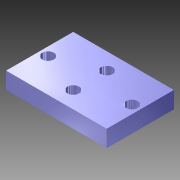
# Autodesk Inventor part: tapa polea x
Saved by Autodesk Inventor 2012 SP2 (Build 160219200, 219)
## iProperties
Created: 2014-07-05
Part Number: tapa polea x
Material: Default
Document SubType Name: Modeling
Designer: Principal
Density: 1 g/cm^3
Author: Principal
Autodesk Inventor part; units mm, degrees
ref_plane "YZ Plane" through (0, 0, 0) normal (1, 0, 0) x (0, 1, 0)
ref_plane "XZ Plane" through (0, 0, 0) normal (0, 1, 0) x (-1, 0, 0)
ref_plane "XY Plane" through (0, 0, 0) normal (0, 0, 1) x (1, 0, 0)
sketch "Boceto1" plane through (0, 0, 0) normal (0, 0, 1) x (1, 0, 0)
  line L0 (-7.9599, 1.191) -> (22.0401, 1.191)
  line L1 (22.0401, 1.191) -> (22.0401, -18.809)
  line L2 (22.0401, -18.809) -> (-7.9599, -18.809)
  line L3 (-7.9599, -18.809) -> (-7.9599, 1.191)
  point P0 (0, 0)
  dimension "d0" = 20
  dimension "d10" = 30
  constraints: 8 end point
  measures "d0" distance between parallel lines of L2 L0
  measures "d10" distance between parallel lines of L1 L3
extrude "Extrusión1" add sketch "Boceto1" along normal blind 5
sketch "Boceto2" plane through (0, 0, 5) normal (0, 0, 1) x (1, 0, 0)
  line L0 (22.0401, 1.191) -> (22.0401, -18.809) projected
  line L1 (-7.9599, -18.809) -> (-7.9599, 1.191) projected
  line L2 (22.0401, -18.809) -> (-7.9599, -18.809) projected
  circle A0 centre (-5.4599, -8.809) radius 1.75
  circle A1 centre (19.5401, -8.809) radius 1.75
  point P0 (0, 0)
  dimension "d3" = 3.5
  dimension "d4" = 2.5
  dimension "d5" = 2.5
  dimension "d6" = 10
  dimension "d7" = 10
  constraints: 2 centre point
  measures "d3" diameter of A0
  measures "d4" distance from line of A0.centre L1
  measures "d5" distance from line of A1.centre L0
  measures "d6" distance from line of A0.centre L2
  measures "d7" distance from line of L2 A1.centre
extrude "Extrusión2" cut sketch "Boceto2" against normal blind 5
sketch "Boceto3" plane through (0, 0, 5) normal (0, 0, 1) x (1, 0, 0)
  line L0 (-7.9599, 1.191) -> (22.0401, 1.191) projected
  line L1 (22.0401, -18.809) -> (-7.9599, -18.809) projected
  circle A0 centre (7.0401, -3.809) radius 1.75
  circle A1 centre (7.0401, -13.809) radius 1.75
  point P0 (0, 0)
  dimension "d11" = 5
  dimension "d12" = 5
  constraints: 2 centre point
  measures "d11" distance from line of A0.centre L0
  measures "d12" distance from line of A1.centre L1
extrude "Extrusión3" cut sketch "Boceto3" against normal blind 5
